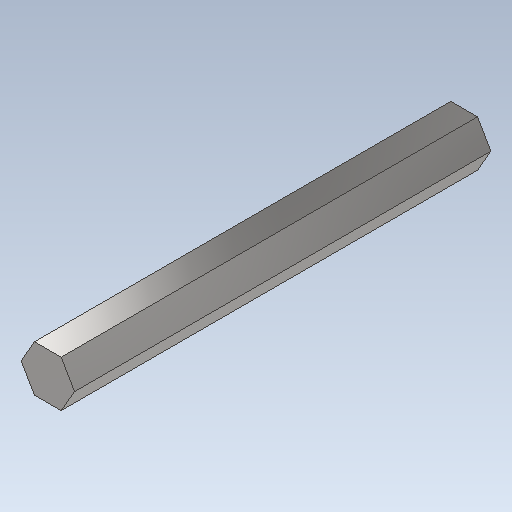
# Autodesk Inventor part: Ch-1-01-0.5x4.5HexShaft
Saved by Autodesk Inventor 2023 (Build 270158000, 158)
## iProperties
Created: 2022-11-08
Part Number: Ch-1-01-0.5x4.5HexShaft
Material: Steel, Alloy
Document SubType Name: Modeling
Designer: megan
Density: 7.73 g/cm^3
Appearance: Semi-Polished
Author: megan
Autodesk Inventor part; units mm, degrees
ref_plane "YZ Plane" through (0, 0, 0) normal (1, 0, 0) x (0, 1, 0)
ref_plane "XZ Plane" through (0, 0, 0) normal (0, 1, 0) x (-1, 0, 0)
ref_plane "XY Plane" through (0, 0, 0) normal (0, 0, 1) x (1, 0, 0)
sketch "Sketch1" plane through (0, 0, 0) normal (0, 0, 1) x (1, 0, 0)
  line L0 (7.3323, 0) -> (3.6662, -6.35)
  line L1 (3.6662, -6.35) -> (-3.6662, -6.35)
  line L2 (-3.6662, -6.35) -> (-7.3323, 0)
  line L3 (-7.3323, 0) -> (-3.6662, 6.35)
  line L4 (-3.6662, 6.35) -> (3.6662, 6.35)
  line L5 (3.6662, 6.35) -> (7.3323, 0)
  point P0 (0, 0)
  point P1 (0, 0)
  dimension "d0" = 12.7
  constraints: 12 end point, 1 coincident, 13 other
  measures "d0" distance between parallel lines of L5 L2
extrude "Extrusion1" add sketch "Sketch1" along normal mid plane 114.3
body "Solid1"
